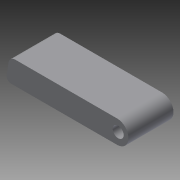
# Autodesk Inventor part: FelixOriginalBearingHolder
Saved by Autodesk Inventor 2015 SP1 (Build 190203100, 203)
## iProperties
Created: 2014-12-14
Part Number: FelixOriginalBearingHolder
Material: Generic
Document SubType Name: Modeling
Designer: Jack
Density: 1 g/cm^3
Appearance: Default
Author: Jack
Autodesk Inventor part; units mm, degrees
ref_plane "YZ Plane" through (0, 0, 0) normal (1, 0, 0) x (0, 1, 0)
ref_plane "XZ Plane" through (0, 0, 0) normal (0, 1, 0) x (-1, 0, 0)
ref_plane "XY Plane" through (0, 0, 0) normal (0, 0, 1) x (1, 0, 0)
sketch "Sketch1" plane through (0, 0, 0) normal (0, 0, 1) x (1, 0, 0)
  line L0 (0, 0) -> (1.4521, 9.38)
  line L1 (1.4521, 9.38) -> (50.35, 9.38)
  line L2 (50.35, 9.38) -> (50.35, 0)
  line L3 (50.35, 0) -> (0, 0)
  dimension "d7" = 81.2
  dimension "d8" = 50.35
  dimension "d9" = 9.38
  constraints: 8 end point, 2 perpendicular, 1 horizontal
  measures "d7" angle of L3 L0
  measures "d8" distance of L2.end L0.start
  measures "d9" distance of L1.end L2.end
extrude "Extrusion1" add sketch "Sketch1" along normal blind 18.5
fillet "Fillet1" radius 2.85 1 edges at (1.4521, 9.38, 9.25)
fillet "Fillet2" radius 1.85 1 edges at (0, 0, 9.25)
sketch "Sketch3" plane through (0, 0, 18.5) normal (0, 0, 1) x (1, 0, 0)
  line L0 (2.1584, 0) -> (50.35, 0) projected
  line L1 (50.35, 0) -> (50.35, 9.38) projected
  circle A0 centre (46.18, 4.8) radius 2.25
  point P0 (0, 0)
  dimension "d13" = 4.5
  dimension "d14" = 4.8
  dimension "d15" = 4.17
  constraints: 1 centre point
  measures "d13" diameter of A0
  measures "d14" distance from line of L0 A0.centre
  measures "d15" distance from line of L1 A0.centre
extrude "Extrusion2" cut sketch "Sketch3" against normal up to next
fillet "Fillet3" radius 4.6 2 edges at (50.35, 9.38, 9.25) (50.35, 0, 9.25)
body "Solid1"
